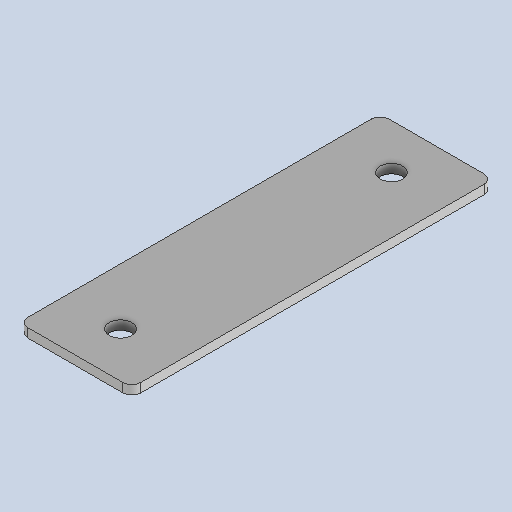
# Autodesk Inventor part: NDM 11.025 bracket 25
Saved by Autodesk Inventor 2025 (Build 290162010, 162A)
## iProperties
Created: 2024-06-12
Part Number: NDM 11.025 bracket 25
Material: Stainless Steel
Document SubType Name: Sheet Metal
Designer: admin
Density: 8 g/cm^3
Flat Pattern Width: 2.5 cm
Flat Pattern Length: 8 cm
Flat Pattern Area: 20 cm^2
Sheet Metal Rule: AISI304 2mm Die16
Sheet Metal Width: 25,000 mm
Sheet Metal Length: 80,000 mm
Sheet Metal Area: 2000,000 mm^2
Appearance: Default
Description: 2mm
Mass: 31.3167 g
Surface Area: 43.9056 cm^2
Volume: 3.91459 cm^3
Author: admin
Revision Number: 60
Autodesk Inventor part; units mm, degrees
ref_plane "YZ Plane" through (0, 0, 0) normal (1, 0, 0) x (0, 1, 0)
ref_plane "XZ Plane" through (0, 0, 0) normal (0, 1, 0) x (-1, 0, 0)
ref_plane "XY Plane" through (0, 0, 0) normal (0, 0, 1) x (1, 0, 0)
sketch "Sketch1" plane through (0, 0, 0) normal (0, 0, 1) x (1, 0, 0)
  line L0 (-12.5, 0) -> (12.5, 0)
  line L1 (12.5, 0) -> (12.5, -80)
  line L2 (12.5, -80) -> (-12.5, -80)
  line L3 (-12.5, -80) -> (-12.5, 0)
  point P0 (0, 0)
  point P1 (0, 0)
  dimension "d0" = 25
  dimension "d1" = 80
  measures "d0" distance of L1.end L2.end
  measures "d1" distance of L0.end L1.end
extrude "Plate1" add sketch "Sketch1" along normal blind 2
sketch "Sketch8" plane through (0, 0, 2) normal (0, 0, 1) x (1, 0, 0)
  line L0 (-12.5, -80) -> (-12.5, 0) construction
  line L1 (12.5, -80) -> (-12.5, -80) projected
  line L2 (12.5, 0) -> (12.5, -80) projected
  line L3 (-12.5, 0) -> (12.5, 0) projected
  circle A0 centre (0, -70) radius 2.5
  circle A1 centre (0, -10) radius 2.5
  line L4 (-12.5, 0) -> (-12.5, -80) construction
  line L5 (-12.5, -40) -> (12.5, -40) construction
  point P0 (0, 0)
  dimension "d34" = 5
  dimension "d35" = 10
  constraints: 2 centre point, 2 end point, 2 midpoint, 1 equal radius, 1 vertical alignment, 1 other
  measures "d34" diameter of A0
  measures "d35" distance from line of L1 A0.centre
extrude "Extrusion3" cut sketch "Sketch8" against normal through all
fillet "Fillet2" radius 2 4 edges at (-12.5, -80, 1) (12.5, -80, 1) (12.5, 0, 1) (-12.5, 0, 1)
equation "\"d2\" = Thickness"
equation "\"BendReliefWidth\" = Thickness"
equation "\"BendReliefDepth\" = 0.5 * Thickness"
equation "\"CornerReliefSize\" = 4 * Thickness"
equation "\"MinimumRemnant\" = 2 * Thickness"
equation "\"TransitionRadius\" = BendRadius"
equation "\"JacobiRadiusSize\" = BendRadius"
equation "\"GapSize\" = Thickness"
equation "\"Thickness\" = 2"
equation "\"BendRadius\" = 2.75"
body "Solid1"
